Autodesk Fusion 360 part; units mm, degrees
(part 6 of 15)
  spline S4 degree 5 poles (-14.2309, -4.8539) (-14.231, -4.8539) (-14.2312, -4.854) (-14.2315, -4.8541) (-14.232, -4.8543) (-14.2328, -4.8546) (-14.2336, -4.8549) (-14.2346, -4.8552) (-14.2356, -4.8556) (-14.2368, -4.8561) (-14.2381, -4.8566) (-14.2395, -4.8571) (-14.241, -4.8577) (-14.2426, -4.8583) (-14.2443, -4.8589) (-14.2461, -4.8596) (-14.2479, -4.8604) (-14.2499, -4.8612) (-14.252, -4.862) (-14.2542, -4.8629) (-14.2564, -4.8638) (-14.2588, -4.8648) (-14.2612, -4.8658) (-14.2637, -4.8669) (-14.2663, -4.868) (-14.269, -4.8691) (-14.2718, -4.8703) (-14.2747, -4.8715) (-14.2776, -4.8728) (-14.2807, -4.8741) (-14.2838, -4.8755) (-14.2869, -4.8769) (-14.2902, -4.8784) (-14.2935, -4.8799) (-14.2969, -4.8814) (-14.3004, -4.883) (-14.304, -4.8846) (-14.3076, -4.8863) (-14.3113, -4.888) (-14.3151, -4.8898) (-14.319, -4.8916) (-14.3229, -4.8935) (-14.3269, -4.8954) (-14.3309, -4.8973) (-14.335, -4.8993) (-14.3392, -4.9014) (-14.3435, -4.9035) (-14.3478, -4.9056) (-14.3521, -4.9078) (-14.3566, -4.91) (-14.3611, -4.9122) (-14.3656, -4.9145) (-14.3703, -4.9169) (-14.375, -4.9193) (-14.3797, -4.9217) (-14.3845, -4.9242) (-14.3894, -4.9268) (-14.3943, -4.9293) (-14.3992, -4.932) (-14.4043, -4.9346) (-14.4094, -4.9373) (-14.4145, -4.9401) (-14.4197, -4.9429) (-14.4249, -4.9457) (-14.4302, -4.9486) (-14.4356, -4.9516) (-14.441, -4.9545) (-14.4465, -4.9576) (-14.452, -4.9606) (-14.4575, -4.9637) (-14.4631, -4.9669) (-14.4688, -4.9701) (-14.4745, -4.9734) (-14.4802, -4.9766) (-14.486, -4.98) (-14.4919, -4.9834) (-14.4978, -4.9868) (-14.5037, -4.9903) (-14.5097, -4.9938) (-14.5157, -4.9974) (-14.5218, -5.001) (-14.5279, -5.0046) (-14.534, -5.0083) (-14.5402, -5.0121) (-14.5465, -5.0158) (-14.5528, -5.0197) (-14.5591, -5.0235) (-14.5655, -5.0275) (-14.5719, -5.0314) (-14.5783, -5.0354) (-14.5848, -5.0395) (-14.5913, -5.0436) (-14.5979, -5.0477) (-14.6045, -5.0519) (-14.6111, -5.0562) (-14.6178, -5.0604) (-14.6245, -5.0648) (-14.6313, -5.0691) (-14.6381, -5.0735) (-14.6449, -5.078) (-14.6518, -5.0825) (-14.6587, -5.087) (-14.6656, -5.0916) (-14.6726, -5.0963) (-14.6796, -5.1009) (-14.6866, -5.1057) (-14.6937, -5.1104) (-14.7008, -5.1152) (-14.7079, -5.1201) (-14.7151, -5.125) (-14.7223, -5.1299) (-14.7295, -5.1349) (-14.7368, -5.14) (-14.7441, -5.145) (-14.7514, -5.1502) (-14.7587, -5.1553) (-14.7661, -5.1605) (-14.7735, -5.1658) (-14.781, -5.1711) (-14.7884, -5.1764) (-14.7959, -5.1818) (-14.8035, -5.1873) (-14.811, -5.1927) (-14.8186, -5.1982) (-14.8262, -5.2038) (-14.8338, -5.2094) (-14.8415, -5.2151) (-14.8492, -5.2208) (-14.8569, -5.2265) (-14.8646, -5.2323) (-14.8724, -5.2381) (-14.8802, -5.244) (-14.888, -5.2499) (-14.8959, -5.2559) (-14.9037, -5.2619) (-14.9116, -5.2679) (-14.9195, -5.274) (-14.9275, -5.2801) (-14.9354, -5.2863) (-14.9434, -5.2925) (-14.9514, -5.2988) (-14.9594, -5.3051) (-14.9675, -5.3114) (-14.9755, -5.3178) (-14.9836, -5.3243) (-14.9918, -5.3308) (-14.9999, -5.3373) (-15.008, -5.3439) (-15.0162, -5.3505) (-15.0244, -5.3571) (-15.0326, -5.3638) (-15.0409, -5.3706) (-15.0491, -5.3773) (-15.0574, -5.3842) (-15.0657, -5.391) (-15.074, -5.398) (-15.0823, -5.4049) (-15.0907, -5.4119) (-15.099, -5.419) (-15.1074, -5.426) (-15.1158, -5.4332) (-15.1242, -5.4403) (-15.1327, -5.4476) (-15.1411, -5.4548) (-15.1496, -5.4621) (-15.1581, -5.4695) (-15.1666, -5.4769) (-15.1751, -5.4843) (-15.1836, -5.4918) (-15.1922, -5.4993) (-15.2008, -5.5068) (-15.2093, -5.5144) (-15.2179, -5.5221) (-15.2265, -5.5298) (-15.2352, -5.5375) (-15.2438, -5.5453) (-15.2524, -5.5531) (-15.2611, -5.5609) (-15.2698, -5.5688) (-15.2785, -5.5768) (-15.2872, -5.5848) (-15.2959, -5.5928) (-15.3046, -5.6008) (-15.3134, -5.609) (-15.3221, -5.6171) (-15.3309, -5.6253) (-15.3397, -5.6335) (-15.3484, -5.6418) (-15.3572, -5.6501) (-15.3661, -5.6585) (-15.3749, -5.6669) (-15.3837, -5.6753) (-15.3926, -5.6838) (-15.4014, -5.6924) (-15.4103, -5.7009) (-15.4192, -5.7096) (-15.428, -5.7182) (-15.4369, -5.7269) (-15.4458, -5.7356) (-15.4548, -5.7444) (-15.4637, -5.7532) (-15.4726, -5.7621) (-15.4816, -5.771) (-15.4905, -5.78) (-15.4995, -5.789) (-15.5084, -5.798) (-15.5174, -5.8071) (-15.5264, -5.8162) (-15.5354, -5.8253) (-15.5444, -5.8345) (-15.5534, -5.8437) (-15.5624, -5.853) (-15.5714, -5.8623) (-15.5804, -5.8717) (-15.5895, -5.8811) (-15.5985, -5.8905) (-15.6075, -5.9) (-15.6166, -5.9096) (-15.6256, -5.9191) (-15.6347, -5.9287) (-15.6438, -5.9384) (-15.6529, -5.9481) (-15.6619, -5.9578) (-15.671, -5.9676) (-15.6801, -5.9774) (-15.6892, -5.9872) (-15.6983, -5.9971) (-15.7074, -6.007) (-15.7165, -6.017) (-15.7256, -6.027) (-15.7347, -6.0371) (-15.7439, -6.0472) (-15.753, -6.0573) (-15.7621, -6.0675) (-15.7712, -6.0777) (-15.7804, -6.0879) (-15.7895, -6.0982) (-15.7986, -6.1086) (-15.8078, -6.1189) (-15.8169, -6.1293) (-15.8261, -6.1398) (-15.8334, -6.1482) (-15.8389, -6.1545) (-15.8425, -6.1587) (-15.8444, -6.1608) knots 0 0 0 0 0 0 0.00416667 0.00833333 0.0125 0.01666667 0.02083333 0.025 0.02916667 0.03333333 0.0375 0.04166667 0.04583333 0.05 0.05416667 0.05833333 0.0625 0.06666667 0.07083333 0.075 0.07916667 0.08333333 0.0875 0.09166667 0.09583333 0.1 0.10416667 0.10833333 0.1125 0.11666667 0.12083333 0.125 0.12916667 0.13333333 0.1375 0.14166667 0.14583333 0.15 0.15416667 0.15833333 0.1625 0.16666667 0.17083333 0.175 0.17916667 0.18333333 0.1875 0.19166667 0.19583333 0.2 0.20416667 0.20833333 0.2125 0.21666667 0.22083333 0.225 0.22916667 0.23333333 0.2375 0.24166667 0.24583333 0.25 0.25416667 0.25833333 0.2625 0.26666667 0.27083333 0.275 0.27916667 0.28333333 0.2875 0.29166667 0.29583333 0.3 0.30416667 0.30833333 0.3125 0.31666667 0.32083333 0.325 0.32916667 0.33333333 0.3375 0.34166667 0.34583333 0.35 0.35416667 0.35833333 0.3625 0.36666667 0.37083333 0.375 0.37916667 0.38333333 0.3875 0.39166667 0.39583333 0.4 0.40416667 0.40833333 0.4125 0.41666667 0.42083333 0.425 0.42916667 0.43333333 0.4375 0.44166667 0.44583333 0.45 0.45416667 0.45833333 0.4625 0.46666667 0.47083333 0.475 0.47916667 0.48333333 0.4875 0.49166667 0.49583333 0.5 0.50416667 0.50833333 0.5125 0.51666667 0.52083333 0.525 0.52916667 0.53333333 0.5375 0.54166667 0.54583333 0.55 0.55416667 0.55833333 0.5625 0.56666667 0.57083333 0.575 0.57916667 0.58333333 0.5875 0.59166667 0.59583333 0.6 0.60416667 0.60833333 0.6125 0.61666667 0.62083333 0.625 0.62916667 0.63333333 0.6375 0.64166667 0.64583333 0.65 0.65416667 0.65833333 0.6625 0.66666667 0.67083333 0.675 0.67916667 0.68333333 0.6875 0.69166667 0.69583333 0.7 0.70416667 0.70833333 0.7125 0.71666667 0.72083333 0.725 0.72916667 0.73333333 0.7375 0.74166667 0.74583333 0.75 0.75416667 0.75833333 0.7625 0.76666667 0.77083333 0.775 0.77916667 0.78333333 0.7875 0.79166667 0.79583333 0.8 0.80416667 0.80833333 0.8125 0.81666667 0.82083333 0.825 0.82916667 0.83333333 0.8375 0.84166667 0.84583333 0.85 0.85416667 0.85833333 0.8625 0.86666667 0.87083333 0.875 0.87916667 0.88333333 0.8875 0.89166667 0.89583333 0.9 0.90416667 0.90833333 0.9125 0.91666667 0.92083333 0.925 0.92916667 0.93333333 0.9375 0.94166667 0.94583333 0.95 0.95416667 0.95833333 0.9625 0.96666667 0.97083333 0.975 0.97916667 0.98333333 0.9875 0.99166667 0.99583333 1 1 1 1 1 1
  arc A5 (-15.8444, -6.1608) -> (-15.56, -6.8473) centre (0, 0) ccw
  spline S5 degree 5 poles (-15.56, -6.8473) (-15.5572, -6.8475) (-15.5517, -6.8479) (-15.5433, -6.8485) (-15.5322, -6.8492) (-15.5184, -6.8502) (-15.5045, -6.851) (-15.4907, -6.8519) (-15.477, -6.8528) (-15.4632, -6.8536) (-15.4495, -6.8544) (-15.4358, -6.8551) (-15.4222, -6.8559) (-15.4086, -6.8566) (-15.395, -6.8573) (-15.3814, -6.8579) (-15.3679, -6.8586) (-15.3544, -6.8592) (-15.341, -6.8598) (-15.3275, -6.8603) (-15.3141, -6.8609) (-15.3008, -6.8614) (-15.2874, -6.8619) (-15.2741, -6.8623) (-15.2609, -6.8628) (-15.2476, -6.8632) (-15.2344, -6.8636) (-15.2213, -6.8639) (-15.2081, -6.8642) (-15.195, -6.8646) (-15.182, -6.8648) (-15.1689, -6.8651) (-15.1559, -6.8653) (-15.143, -6.8656) (-15.13, -6.8657) (-15.1171, -6.8659) (-15.1043, -6.866) (-15.0915, -6.8662) (-15.0787, -6.8663) (-15.0659, -6.8663) (-15.0532, -6.8664) (-15.0405, -6.8664) (-15.0278, -6.8664) (-15.0152, -6.8664) (-15.0026, -6.8663) (-14.9901, -6.8662) (-14.9776, -6.8661) (-14.9651, -6.866) (-14.9527, -6.8659) (-14.9403, -6.8657) (-14.9279, -6.8655) (-14.9156, -6.8653) (-14.9033, -6.8651) (-14.891, -6.8649) (-14.8788, -6.8646) (-14.8666, -6.8643) (-14.8545, -6.864) (-14.8424, -6.8636) (-14.8303, -6.8633) (-14.8183, -6.8629) (-14.8063, -6.8625) (-14.7943, -6.8621) (-14.7824, -6.8616) (-14.7705, -6.8611) (-14.7587, -6.8606) (-14.7469, -6.8601) (-14.7351, -6.8596) (-14.7234, -6.8591) (-14.7117, -6.8585) (-14.7001, -6.8579) (-14.6885, -6.8573) (-14.6769, -6.8567) (-14.6654, -6.856) (-14.6539, -6.8553) (-14.6425, -6.8546) (-14.6311, -6.8539) (-14.6197, -6.8532) (-14.6084, -6.8524) (-14.5971, -6.8517) (-14.5859, -6.8509) (-14.5747, -6.8501) (-14.5635, -6.8493) (-14.5524, -6.8484) (-14.5414, -6.8475) (-14.5303, -6.8467) (-14.5194, -6.8458) (-14.5084, -6.8449) (-14.4975, -6.8439) (-14.4867, -6.843) (-14.4759, -6.842) (-14.4651, -6.841) (-14.4544, -6.84) (-14.4437, -6.839) (-14.4331, -6.8379) (-14.4225, -6.8369) (-14.4119, -6.8358) (-14.4014, -6.8347) (-14.391, -6.8336) (-14.3805, -6.8325) (-14.3702, -6.8314) (-14.3599, -6.8302) (-14.3496, -6.829) (-14.3394, -6.8278) (-14.3292, -6.8266) (-14.319, -6.8254) (-14.309, -6.8242) (-14.2989, -6.823) (-14.2889, -6.8217) (-14.279, -6.8204) (-14.2691, -6.8191) (-14.2592, -6.8178) (-14.2494, -6.8165) (-14.2397, -6.8152) (-14.2299, -6.8138) (-14.2203, -6.8125) (-14.2107, -6.8111) (-14.2011, -6.8097) (-14.1916, -6.8083) (-14.1821, -6.8069) (-14.1727, -6.8055) (-14.1634, -6.8041) (-14.154, -6.8026) (-14.1448, -6.8011) (-14.1356, -6.7997) (-14.1264, -6.7982) (-14.1173, -6.7967) (-14.1082, -6.7952) (-14.0992, -6.7937) (-14.0903, -6.7922) (-14.0814, -6.7906) (-14.0725, -6.7891) (-14.0637, -6.7875) (-14.055, -6.786) (-14.0463, -6.7844) (-14.0376, -6.7828) (-14.0291, -6.7812) (-14.0205, -6.7796) (-14.012, -6.778) (-14.0036, -6.7764) (-13.9953, -6.7747) (-13.9869, -6.7731) (-13.9787, -6.7715) (-13.9705, -6.7698) (-13.9623, -6.7682) (-13.9542, -6.7665) (-13.9462, -6.7648) (-13.9382, -6.7632) (-13.9303, -6.7615) (-13.9224, -6.7598) (-13.9146, -6.7581) (-13.9069, -6.7564) (-13.8992, -6.7547) (-13.8916, -6.753) (-13.884, -6.7513) (-13.8765, -6.7496) (-13.869, -6.7478) (-13.8616, -6.7461) (-13.8543, -6.7444) (-13.847, -6.7427) (-13.8398, -6.7409) (-13.8327, -6.7392) (-13.8256, -6.7374) (-13.8185, -6.7357) (-13.8116, -6.734) (-13.8047, -6.7322) (-13.7978, -6.7305) (-13.791, -6.7287) (-13.7843, -6.727) (-13.7777, -6.7253) (-13.7711, -6.7235) (-13.7645, -6.7218) (-13.7581, -6.72) (-13.7517, -6.7183) (-13.7454, -6.7166) (-13.7391, -6.7148) (-13.7329, -6.7131) (-13.7268, -6.7114) (-13.7207, -6.7097) (-13.7147, -6.7079) (-13.7088, -6.7062) (-13.7029, -6.7045) (-13.6971, -6.7028) (-13.6914, -6.7011) (-13.6858, -6.6994) (-13.6802, -6.6977) (-13.6747, -6.6961) (-13.6692, -6.6944) (-13.6639, -6.6927) (-13.6586, -6.6911) (-13.6533, -6.6894) (-13.6482, -6.6878) (-13.6431, -6.6862) (-13.6381, -6.6845) (-13.6332, -6.6829) (-13.6283, -6.6813) (-13.6235, -6.6798) (-13.6188, -6.6782) (-13.6142, -6.6766) (-13.6096, -6.6751) (-13.6051, -6.6736) (-13.6007, -6.672) (-13.5964, -6.6705) (-13.5922, -6.669) (-13.588, -6.6676) (-13.5839, -6.6661) (-13.5799, -6.6647) (-13.576, -6.6633) (-13.5722, -6.6619) (-13.5684, -6.6605) (-13.5647, -6.6591) (-13.5611, -6.6578) (-13.5576, -6.6565) (-13.5542, -6.6552) (-13.5509, -6.6539) (-13.5476, -6.6526) (-13.5445, -6.6514) (-13.5414, -6.6502) (-13.5384, -6.649) (-13.5355, -6.6479) (-13.5327, -6.6468) (-13.53, -6.6457) (-13.5274, -6.6446) (-13.5248, -6.6436) (-13.5224, -6.6426) (-13.5201, -6.6416) (-13.5178, -6.6406) (-13.5156, -6.6397) (-13.5136, -6.6389) (-13.5116, -6.638) (-13.5098, -6.6372) (-13.508, -6.6364) (-13.5063, -6.6357) (-13.5048, -6.635) (-13.5033, -6.6344) (-13.502, -6.6338) (-13.5007, -6.6332) (-13.4996, -6.6327) (-13.4985, -6.6322) (-13.4976, -6.6318) (-13.4968, -6.6314) (-13.4961, -6.6311) (-13.4956, -6.6308) (-13.4953, -6.6307) (-13.4951, -6.6306) (-13.495, -6.6306) knots -1 -1 -1 -1 -1 -1 -0.99583333 -0.99166667 -0.9875 -0.98333333 -0.97916667 -0.975 -0.97083333 -0.96666667 -0.9625 -0.95833333 -0.95416667 -0.95 -0.94583333 -0.94166667 -0.9375 -0.93333333 -0.92916667 -0.925 -0.92083333 -0.91666667 -0.9125 -0.90833333 -0.90416667 -0.9 -0.89583333 -0.89166667 -0.8875 -0.88333333 -0.87916667 -0.875 -0.87083333 -0.86666667 -0.8625 -0.85833333 -0.85416667 -0.85 -0.84583333 -0.84166667 -0.8375 -0.83333333 -0.82916667 -0.825 -0.82083333 -0.81666667 -0.8125 -0.80833333 -0.80416667 -0.8 -0.79583333 -0.79166667 -0.7875 -0.78333333 -0.77916667 -0.775 -0.77083333 -0.76666667 -0.7625 -0.75833333 -0.75416667 -0.75 -0.74583333 -0.74166667 -0.7375 -0.73333333 -0.72916667 -0.725 -0.72083333 -0.71666667 -0.7125 -0.70833333 -0.70416667 -0.7 -0.69583333 -0.69166667 -0.6875 -0.68333333 -0.67916667 -0.675 -0.67083333 -0.66666667 -0.6625 -0.65833333 -0.65416667 -0.65 -0.64583333 -0.64166667 -0.6375 -0.63333333 -0.62916667 -0.625 -0.62083333 -0.61666667 -0.6125 -0.60833333 -0.60416667 -0.6 -0.59583333 -0.59166667 -0.5875 -0.58333333 -0.57916667 -0.575 -0.57083333 -0.56666667 -0.5625 -0.55833333 -0.55416667 -0.55 -0.54583333 -0.54166667 -0.5375 -0.53333333 -0.52916667 -0.525 -0.52083333 -0.51666667 -0.5125 -0.50833333 -0.50416667 -0.5 -0.49583333 -0.49166667 -0.4875 -0.48333333 -0.47916667 -0.475 -0.47083333 -0.46666667 -0.4625 -0.45833333 -0.45416667 -0.45 -0.44583333 -0.44166667 -0.4375 -0.43333333 -0.42916667 -0.425 -0.42083333 -0.41666667 -0.4125 -0.40833333 -0.40416667 -0.4 -0.39583333 -0.39166667 -0.3875 -0.38333333 -0.37916667 -0.375 -0.37083333 -0.36666667 -0.3625 -0.35833333 -0.35416667 -0.35 -0.34583333 -0.34166667 -0.3375 -0.33333333 -0.32916667 -0.325 -0.32083333 -0.31666667 -0.3125 -0.30833333 -0.30416667 -0.3 -0.29583333 -0.29166667 -0.2875 -0.28333333 -0.27916667 -0.275 -0.27083333 -0.26666667 -0.2625 -0.25833333 -0.25416667 -0.25 -0.24583333 -0.24166667 -0.2375 -0.23333333 -0.22916667 -0.225 -0.22083333 -0.21666667 -0.2125 -0.20833333 -0.20416667 -0.2 -0.19583333 -0.19166667 -0.1875 -0.18333333 -0.17916667 -0.175 -0.17083333 -0.16666667 -0.1625 -0.15833333 -0.15416667 -0.15 -0.14583333 -0.14166667 -0.1375 -0.13333333 -0.12916667 -0.125 -0.12083333 -0.11666667 -0.1125 -0.10833333 -0.10416667 -0.1 -0.09583333 -0.09166667 -0.0875 -0.08333333 -0.07916667 -0.075 -0.07083333 -0.06666667 -0.0625 -0.05833333 -0.05416667 -0.05 -0.04583333 -0.04166667 -0.0375 -0.03333333 -0.02916667 -0.025 -0.02083333 -0.01666667 -0.0125 -0.00833333 -0.00416667 0 0 0 0 0 0
  line L10 (-13.495, -6.6306) -> (-13.4942, -6.6302)
  line L11 (-13.4942, -6.6302) -> (-13.2384, -6.5045)
  arc A6 (-13.2384, -6.5045) -> (-12.7631, -7.3936) centre (0, 0) ccw
  line L12 (-12.7631, -7.3936) -> (-13.0098, -7.5365)
  line L13 (-13.0098, -7.5365) -> (-13.0105, -7.537)
  spline S6 degree 5 poles (-13.0105, -7.537) (-13.0106, -7.537) (-13.0108, -7.5371) (-13.0111, -7.5373) (-13.0115, -7.5376) (-13.0122, -7.538) (-13.013, -7.5384) (-13.0139, -7.539) (-13.0148, -7.5396) (-13.0159, -7.5402) (-13.0171, -7.541) (-13.0183, -7.5417) (-13.0197, -7.5426) (-13.0211, -7.5435) (-13.0226, -7.5445) (-13.0243, -7.5455) (-13.026, -7.5466) (-13.0278, -7.5478) (-13.0296, -7.549) (-13.0316, -7.5503) (-13.0336, -7.5516) (-13.0357, -7.5531) (-13.0379, -7.5545) (-13.0402, -7.5561) (-13.0425, -7.5576) (-13.045, -7.5593) (-13.0474, -7.561) (-13.05, -7.5628) (-13.0526, -7.5646) (-13.0554, -7.5665) (-13.0581, -7.5684) (-13.061, -7.5704) (-13.0639, -7.5725) (-13.0669, -7.5746) (-13.0699, -7.5768) (-13.073, -7.5791) (-13.0762, -7.5814) (-13.0794, -7.5837) (-13.0827, -7.5861) (-13.0861, -7.5886) (-13.0895, -7.5911) (-13.093, -7.5937) (-13.0965, -7.5964) (-13.1001, -7.5991) (-13.1038, -7.6018) (-13.1075, -7.6046) (-13.1112, -7.6075) (-13.115, -7.6104) (-13.1189, -7.6134) (-13.1228, -7.6165) (-13.1268, -7.6196) (-13.1308, -7.6227) (-13.1349, -7.6259) (-13.139, -7.6292) (-13.1432, -7.6325) (-13.1474, -7.6359) (-13.1517, -7.6393) (-13.156, -7.6428) (-13.1604, -7.6463) (-13.1648, -7.6499) (-13.1693, -7.6536) (-13.1738, -7.6573) (-13.1783, -7.6611) (-13.1829, -7.6649) (-13.1875, -7.6687) (-13.1922, -7.6727) (-13.1969, -7.6766) (-13.2017, -7.6807) (-13.2065, -7.6847) (-13.2113, -7.6889) (-13.2162, -7.6931) (-13.2211, -7.6973) (-13.2261, -7.7016) (-13.2311, -7.706) (-13.2361, -7.7104) (-13.2412, -7.7148) (-13.2463, -7.7194) (-13.2515, -7.7239) (-13.2566, -7.7285) (-13.2618, -7.7332) (-13.2671, -7.7379) (-13.2724, -7.7427) (-13.2777, -7.7475) (-13.2831, -7.7524) (-13.2884, -7.7573) (-13.2939, -7.7623) (-13.2993, -7.7674) (-13.3048, -7.7724) (-13.3103, -7.7776) (-13.3158, -7.7828) (-13.3214, -7.788) (-13.327, -7.7933) (-13.3326, -7.7987) (-13.3383, -7.8041) (-13.344, -7.8095) (-13.3497, -7.815) (-13.3555, -7.8206) (-13.3612, -7.8262) (-13.367, -7.8318) (-13.3728, -7.8375) (-13.3787, -7.8433) (-13.3846, -7.8491) (-13.3905, -7.8549) (-13.3964, -7.8608) (-13.4024, -7.8668) (-13.4083, -7.8728) (-13.4143, -7.8788) (-13.4204, -7.8849) (-13.4264, -7.8911) (-13.4325, -7.8973) (-13.4386, -7.9035) (-13.4447, -7.9099) (-13.4508, -7.9162) (-13.457, -7.9226) (-13.4632, -7.9291) (-13.4694, -7.9356) (-13.4756, -7.9421) (-13.4819, -7.9487) (-13.4881, -7.9554) (-13.4944, -7.9621) (-13.5007, -7.9688) (-13.507, -7.9756) (-13.5134, -7.9824) (-13.5197, -7.9893) (-13.5261, -7.9963) (-13.5325, -8.0033) (-13.5389, -8.0103) (-13.5453, -8.0174) (-13.5518, -8.0245) (-13.5583, -8.0317) (-13.5647, -8.0389) (-13.5712, -8.0462) (-13.5777, -8.0535) (-13.5843, -8.0609) (-13.5908, -8.0683) (-13.5974, -8.0758) (-13.6039, -8.0833) (-13.6105, -8.0909) (-13.6171, -8.0985) (-13.6237, -8.1061) (-13.6304, -8.1138) (-13.637, -8.1216) (-13.6437, -8.1294) (-13.6503, -8.1372) (-13.657, -8.1451) (-13.6637, -8.1531) (-13.6704, -8.1611) (-13.6771, -8.1691) (-13.6839, -8.1772) (-13.6906, -8.1853) (-13.6973, -8.1935) (-13.7041, -8.2017) (-13.7109, -8.21) (-13.7177, -8.2183) (-13.7245, -8.2266) (-13.7313, -8.235) (-13.7381, -8.2435) (-13.7449, -8.252) (-13.7517, -8.2605) (-13.7586, -8.2691) (-13.7654, -8.2777) (-13.7723, -8.2864) (-13.7791, -8.2951) (-13.786, -8.3039) (-13.7929, -8.3127) (-13.7998, -8.3216) (-13.8067, -8.3305) (-13.8136, -8.3394) (-13.8205, -8.3484) (-13.8274, -8.3575) (-13.8343, -8.3665) (-13.8413, -8.3757) (-13.8482, -8.3848) (-13.8552, -8.3941) (-13.8621, -8.4033) (-13.8691, -8.4126) (-13.876, -8.422) (-13.883, -8.4314) (-13.89, -8.4408) (-13.8969, -8.4503) (-13.9039, -8.4598) (-13.9109, -8.4694) (-13.9179, -8.479) (-13.9249, -8.4887) (-13.9319, -8.4984) (-13.9389, -8.5081) (-13.9459, -8.5179) (-13.9529, -8.5277) (-13.9599, -8.5376) (-13.9669, -8.5475) (-13.9739, -8.5575) (-13.9809, -8.5675) (-13.9879, -8.5776) (-13.995, -8.5877) (-14.002, -8.5978) (-14.009, -8.608) (-14.016, -8.6182) (-14.0231, -8.6285) (-14.0301, -8.6388) (-14.0371, -8.6491) (-14.0441, -8.6595) (-14.0512, -8.67) (-14.0582, -8.6804) (-14.0652, -8.6909) (-14.0723, -8.7015) (-14.0793, -8.7121) (-14.0863, -8.7228) (-14.0934, -8.7335) (-14.1004, -8.7442) (-14.1074, -8.755) (-14.1145, -8.7658) (-14.1215, -8.7766) (-14.1285, -8.7875) (-14.1355, -8.7985) (-14.1426, -8.8095) (-14.1496, -8.8205) (-14.1566, -8.8315) (-14.1636, -8.8426) (-14.1706, -8.8538) (-14.1777, -8.865) (-14.1847, -8.8762) (-14.1917, -8.8875) (-14.1987, -8.8988) (-14.2057, -8.9101) (-14.2127, -8.9215) (-14.2197, -8.933) (-14.2267, -8.9445) (-14.2337, -8.956) (-14.2407, -8.9675) (-14.2476, -8.9791) (-14.2546, -8.9908) (-14.2616, -9.0024) (-14.2686, -9.0142) (-14.2755, -9.0259) (-14.2825, -9.0377) (-14.2895, -9.0495) (-14.2964, -9.0614) (-14.3033, -9.0733) (-14.3103, -9.0853) (-14.3172, -9.0973) (-14.3242, -9.1093) (-14.3297, -9.119) (-14.3339, -9.1263) (-14.3366, -9.1311) (-14.338, -9.1335) knots 0 0 0 0 0 0 0.00416667 0.00833333 0.0125 0.01666667 0.02083333 0.025 0.02916667 0.03333333 0.0375 0.04166667 0.04583333 0.05 0.05416667 0.05833333 0.0625 0.06666667 0.07083333 0.075 0.07916667 0.08333333 0.0875 0.09166667 0.09583333 0.1 0.10416667 0.10833333 0.1125 0.11666667 0.12083333 0.125 0.12916667 0.13333333 0.1375 0.14166667 0.14583333 0.15 0.15416667 0.15833333 0.1625 0.16666667 0.17083333 0.175 0.17916667 0.18333333 0.1875 0.19166667 0.19583333 0.2 0.20416667 0.20833333 0.2125 0.21666667 0.22083333 0.225 0.22916667 0.23333333 0.2375 0.24166667 0.24583333 0.25 0.25416667 0.25833333 0.2625 0.26666667 0.27083333 0.275 0.27916667 0.28333333 0.2875 0.29166667 0.29583333 0.3 0.30416667 0.30833333 0.3125 0.31666667 0.32083333 0.325 0.32916667 0.33333333 0.3375 0.34166667 0.34583333 0.35 0.35416667 0.35833333 0.3625 0.36666667 0.37083333 0.375 0.37916667 0.38333333 0.3875 0.39166667 0.39583333 0.4 0.40416667 0.40833333 0.4125 0.41666667 0.42083333 0.425 0.42916667 0.43333333 0.4375 0.44166667 0.44583333 0.45 0.45416667 0.45833333 0.4625 0.46666667 0.47083333 0.475 0.47916667 0.48333333 0.4875 0.49166667 0.49583333 0.5 0.50416667 0.50833333 0.5125 0.51666667 0.52083333 0.525 0.52916667 0.53333333 0.5375 0.54166667 0.54583333 0.55 0.55416667 0.55833333 0.5625 0.56666667 0.57083333 0.575 0.57916667 0.58333333 0.5875 0.59166667 0.59583333 0.6 0.60416667 0.60833333 0.6125 0.61666667 0.62083333 0.625 0.62916667 0.63333333 0.6375 0.64166667 0.64583333 0.65 0.65416667 0.65833333 0.6625 0.66666667 0.67083333 0.675 0.67916667 0.68333333 0.6875 0.69166667 0.69583333 0.7 0.70416667 0.70833333 0.7125 0.71666667 0.72083333 0.725 0.72916667 0.73333333 0.7375 0.74166667 0.74583333 0.75 0.75416667 0.75833333 0.7625 0.76666667 0.77083333 0.775 0.77916667 0.78333333 0.7875 0.79166667 0.79583333 0.8 0.80416667 0.80833333 0.8125 0.81666667 0.82083333 0.825 0.82916667 0.83333333 0.8375 0.84166667 0.84583333 0.85 0.85416667 0.85833333 0.8625 0.86666667 0.87083333 0.875 0.87916667 0.88333333 0.8875 0.89166667 0.89583333 0.9 0.90416667 0.90833333 0.9125 0.91666667 0.92083333 0.925 0.92916667 0.93333333 0.9375 0.94166667 0.94583333 0.95 0.95416667 0.95833333 0.9625 0.96666667 0.97083333 0.975 0.97916667 0.98333333 0.9875 0.99166667 0.99583333 1 1 1 1 1 1
  arc A7 (-14.338, -9.1335) -> (-13.9252, -9.7513) centre (0, 0) ccw
  spline S7 degree 5 poles (-13.9252, -9.7513) (-13.9224, -9.751) (-13.9169, -9.7503) (-13.9086, -9.7492) (-13.8975, -9.7478) (-13.8838, -9.746) (-13.87, -9.7442) (-13.8563, -9.7424) (-13.8427, -9.7405) (-13.829, -9.7386) (-13.8154, -9.7367) (-13.8019, -9.7348) (-13.7883, -9.7329) (-13.7748, -9.7309) (-13.7614, -9.7289) (-13.748, -9.7269) (-13.7346, -9.7249) (-13.7212, -9.7229) (-13.7079, -9.7208) (-13.6946, -9.7188) (-13.6814, -9.7167) (-13.6682, -9.7146) (-13.655, -9.7125) (-13.6419, -9.7103) (-13.6288, -9.7081) (-13.6157, -9.706) (-13.6027, -9.7038) (-13.5897, -9.7015) (-13.5768, -9.6993) (-13.5639, -9.6971) (-13.551, -9.6948) (-13.5382, -9.6925) (-13.5254, -9.6902) (-13.5126, -9.6879) (-13.4999, -9.6855) (-13.4872, -9.6832) (-13.4746, -9.6808) (-13.462, -9.6784) (-13.4494, -9.676) (-13.4369, -9.6736) (-13.4244, -9.6712) (-13.4119, -9.6687) (-13.3995, -9.6662) (-13.3871, -9.6637) (-13.3748, -9.6612) (-13.3625, -9.6587) (-13.3503, -9.6562) (-13.3381, -9.6536) (-13.3259, -9.6511) (-13.3137, -9.6485) (-13.3017, -9.6459) (-13.2896, -9.6433) (-13.2776, -9.6407) (-13.2656, -9.638) (-13.2537, -9.6354) (-13.2418, -9.6327) (-13.2299, -9.63) (-13.2181, -9.6273) (-13.2064, -9.6246) (-13.1946, -9.6219) (-13.183, -9.6192) (-13.1713, -9.6164) (-13.1597, -9.6137) (-13.1482, -9.6109) (-13.1367, -9.6081) (-13.1252, -9.6053) (-13.1137, -9.6025) (-13.1024, -9.5997) (-13.091, -9.5968) (-13.0797, -9.594) (-13.0685, -9.5911) (-13.0572, -9.5882) (-13.0461, -9.5853) (-13.0349, -9.5824) (-13.0238, -9.5795) (-13.0128, -9.5766) (-13.0018, -9.5737) (-12.9909, -9.5707) (-12.9799, -9.5678) (-12.9691, -9.5648) (-12.9583, -9.5618) (-12.9475, -9.5589) (-12.9368, -9.5559) (-12.9261, -9.5529) (-12.9154, -9.5498) (-12.9048, -9.5468) (-12.8943, -9.5438) (-12.8838, -9.5407) (-12.8733, -9.5377) (-12.8629, -9.5346) (-12.8525, -9.5316) (-12.8422, -9.5285) (-12.8319, -9.5254) (-12.8217, -9.5223) (-12.8115, -9.5192) (-12.8014, -9.5161) (-12.7913, -9.513) (-12.7813, -9.5098) (-12.7713, -9.5067) (-12.7613, -9.5036) (-12.7514, -9.5004) (-12.7416, -9.4973) (-12.7318, -9.4941) (-12.722, -9.491) (-12.7123, -9.4878) (-12.7027, -9.4846) (-12.6931, -9.4814) (-12.6835, -9.4782) (-12.674, -9.4751) (-12.6645, -9.4719) (-12.6551, -9.4687) (-12.6458, -9.4655) (-12.6365, -9.4622) (-12.6272, -9.459) (-12.618, -9.4558) (-12.6088, -9.4526) (-12.5997, -9.4494) (-12.5907, -9.4461) (-12.5817, -9.4429) (-12.5727, -9.4397) (-12.5638, -9.4364) (-12.555, -9.4332) (-12.5462, -9.43) (-12.5374, -9.4267) (-12.5287, -9.4235) (-12.5201, -9.4203) (-12.5115, -9.417) (-12.5029, -9.4138) (-12.4944, -9.4105) (-12.486, -9.4073) (-12.4776, -9.404) (-12.4693, -9.4008) (-12.461, -9.3976) (-12.4528, -9.3943) (-12.4447, -9.3911) (-12.4365, -9.3878) (-12.4285, -9.3846) (-12.4205, -9.3814) (-12.4125, -9.3781) (-12.4046, -9.3749) (-12.3968, -9.3717) (-12.389, -9.3685) (-12.3813, -9.3652) (-12.3736, -9.362) (-12.366, -9.3588) (-12.3585, -9.3556) (-12.351, -9.3524) (-12.3435, -9.3492) (-12.3362, -9.346) (-12.3288, -9.3428) (-12.3216, -9.3397) (-12.3144, -9.3365) (-12.3072, -9.3333) (-12.3001, -9.3302) (-12.2931, -9.327) (-12.2861, -9.3239) (-12.2792, -9.3208) (-12.2723, -9.3176) (-12.2655, -9.3145) (-12.2588, -9.3114) (-12.2521, -9.3083) (-12.2455, -9.3052) (-12.2389, -9.3021) (-12.2324, -9.2991) (-12.226, -9.296) (-12.2196, -9.293) (-12.2133, -9.2899) (-12.2071, -9.2869) (-12.2009, -9.2839) (-12.1948, -9.2809) (-12.1887, -9.278) (-12.1827, -9.275) (-12.1768, -9.272) (-12.1709, -9.2691) (-12.1651, -9.2662) (-12.1594, -9.2633) (-12.1537, -9.2604) (-12.1481, -9.2575) (-12.1425, -9.2547) (-12.1371, -9.2518) (-12.1316, -9.249) (-12.1263, -9.2462) (-12.121, -9.2434) (-12.1158, -9.2407) (-12.1107, -9.2379) (-12.1056, -9.2352) (-12.1006, -9.2325) (-12.0956, -9.2298) (-12.0907, -9.2272) (-12.0859, -9.2245) (-12.0812, -9.2219) (-12.0765, -9.2193) (-12.0719, -9.2168) (-12.0674, -9.2142) (-12.063, -9.2117) (-12.0586, -9.2092) (-12.0543, -9.2068) (-12.05, -9.2043) (-12.0459, -9.2019) (-12.0418, -9.1996) (-12.0378, -9.1972) (-12.0338, -9.1949) (-12.0299, -9.1926) (-12.0261, -9.1904) (-12.0224, -9.1881) (-12.0188, -9.1859) (-12.0152, -9.1838) (-12.0117, -9.1817) (-12.0083, -9.1796) (-12.005, -9.1775) (-12.0017, -9.1755) (-11.9985, -9.1735) (-11.9954, -9.1716) (-11.9924, -9.1697) (-11.9895, -9.1678) (-11.9866, -9.166) (-11.9838, -9.1642) (-11.9811, -9.1625) (-11.9785, -9.1608) (-11.976, -9.1591) (-11.9735, -9.1575) (-11.9711, -9.156) (-11.9689, -9.1545) (-11.9667, -9.153) (-11.9646, -9.1516) (-11.9625, -9.1502) (-11.9606, -9.1489) (-11.9588, -9.1477) (-11.957, -9.1465) (-11.9553, -9.1453) (-11.9537, -9.1442) (-11.9523, -9.1432) (-11.9509, -9.1422) (-11.9496, -9.1413) (-11.9483, -9.1404) (-11.9472, -9.1396) (-11.9462, -9.1389) (-11.9453, -9.1382) (-11.9445, -9.1376) (-11.9437, -9.1371) (-11.9431, -9.1366) (-11.9427, -9.1363) (-11.9424, -9.1361) (-11.9422, -9.136) (-11.9422, -9.1359) knots -1 -1 -1 -1 -1 -1 -0.99583333 -0.99166667 -0.9875 -0.98333333 -0.97916667 -0.975 -0.97083333 -0.96666667 -0.9625 -0.95833333 -0.95416667 -0.95 -0.94583333 -0.94166667 -0.9375 -0.93333333 -0.92916667 -0.925 -0.92083333 -0.91666667 -0.9125 -0.90833333 -0.90416667 -0.9 -0.89583333 -0.89166667 -0.8875 -0.88333333 -0.87916667 -0.875 -0.87083333 -0.86666667 -0.8625 -0.85833333 -0.85416667 -0.85 -0.84583333 -0.84166667 -0.8375 -0.83333333 -0.82916667 -0.825 -0.82083333 -0.81666667 -0.8125 -0.80833333 -0.80416667 -0.8 -0.79583333 -0.79166667 -0.7875 -0.78333333 -0.77916667 -0.775 -0.77083333 -0.76666667 -0.7625 -0.75833333 -0.75416667 -0.75 -0.74583333 -0.74166667 -0.7375 -0.73333333 -0.72916667 -0.725 -0.72083333 -0.71666667 -0.7125 -0.70833333 -0.70416667 -0.7 -0.69583333 -0.69166667 -0.6875 -0.68333333 -0.67916667 -0.675 -0.67083333 -0.66666667 -0.6625 -0.65833333 -0.65416667 -0.65 -0.64583333 -0.64166667 -0.6375 -0.63333333 -0.62916667 -0.625 -0.62083333 -0.61666667 -0.6125 -0.60833333 -0.60416667 -0.6 -0.59583333 -0.59166667 -0.5875 -0.58333333 -0.57916667 -0.575 -0.57083333 -0.56666667 -0.5625 -0.55833333 -0.55416667 -0.55 -0.54583333 -0.54166667 -0.5375 -0.53333333 -0.52916667 -0.525 -0.52083333 -0.51666667 -0.5125 -0.50833333 -0.50416667 -0.5 -0.49583333 -0.49166667 -0.4875 -0.48333333 -0.47916667 -0.475 -0.47083333 -0.46666667 -0.4625 -0.45833333 -0.45416667 -0.45 -0.44583333 -0.44166667 -0.4375 -0.43333333 -0.42916667 -0.425 -0.42083333 -0.41666667 -0.4125 -0.40833333 -0.40416667 -0.4 -0.39583333 -0.39166667 -0.3875 -0.38333333 -0.37916667 -0.375 -0.37083333 -0.36666667 -0.3625 -0.35833333 -0.35416667 -0.35 -0.34583333 -0.34166667 -0.3375 -0.33333333 -0.32916667 -0.325 -0.32083333 -0.31666667 -0.3125 -0.30833333 -0.30416667 -0.3 -0.29583333 -0.29166667 -0.2875 -0.28333333 -0.27916667 -0.275 -0.27083333 -0.26666667 -0.2625 -0.25833333 -0.25416667 -0.25 -0.24583333 -0.24166667 -0.2375 -0.23333333 -0.22916667 -0.225 -0.22083333 -0.21666667 -0.2125 -0.20833333 -0.20416667 -0.2 -0.19583333 -0.19166667 -0.1875 -0.18333333 -0.17916667 -0.175 -0.17083333 -0.16666667 -0.1625 -0.15833333 -0.15416667 -0.15 -0.14583333 -0.14166667 -0.1375 -0.13333333 -0.12916667 -0.125 -0.12083333 -0.11666667 -0.1125 -0.10833333 -0.10416667 -0.1 -0.09583333 -0.09166667 -0.0875 -0.08333333 -0.07916667 -0.075 -0.07083333 -0.06666667 -0.0625 -0.05833333 -0.05416667 -0.05 -0.04583333 -0.04166667 -0.0375 -0.03333333 -0.02916667 -0.025 -0.02083333 -0.01666667 -0.0125 -0.00833333 -0.00416667 0 0 0 0 0 0
  line L14 (-11.9422, -9.1359) -> (-11.9415, -9.1354)
  line L15 (-11.9415, -9.1354) -> (-11.715, -8.9622)
  arc A8 (-11.715, -8.9622) -> (-11.0754, -9.7415) centre (0, 0) ccw
  line L16 (-11.0754, -9.7415) -> (-11.2895, -9.9298)
  line L17 (-11.2895, -9.9298) -> (-11.2902, -9.9304)
  spline S8 degree 5 poles (-11.2902, -9.9304) (-11.2902, -9.9304) (-11.2904, -9.9306) (-11.2906, -9.9308) (-11.291, -9.9312) (-11.2916, -9.9317) (-11.2923, -9.9323) (-11.293, -9.933) (-11.2939, -9.9338) (-11.2948, -9.9346) (-11.2958, -9.9356) (-11.2969, -9.9366) (-11.298, -9.9377) (-11.2993, -9.9389) (-11.3006, -9.9401) (-11.3019, -9.9414) (-11.3034, -9.9429) (-11.3049, -9.9443) (-11.3065, -9.9459) (-11.3082, -9.9476) (-11.3099, -9.9493) (-11.3117, -9.9511) (-11.3136, -9.9529) (-11.3155, -9.9549) (-11.3175, -9.9569) (-11.3196, -9.959) (-11.3217, -9.9612) (-11.3238, -9.9634) (-11.3261, -9.9657) (-11.3284, -9.9681) (-11.3307, -9.9705) (-11.3331, -9.9731) (-11.3355, -9.9756) (-11.3381, -9.9783) (-11.3406, -9.981) (-11.3432, -9.9838) (-11.3459, -9.9867) (-11.3486, -9.9897) (-11.3514, -9.9927) (-11.3542, -9.9958) (-11.357, -9.9989) (-11.3599, -10.0021) (-11.3629, -10.0054) (-11.3659, -10.0088) (-11.3689, -10.0122) (-11.372, -10.0157) (-11.3751, -10.0192) (-11.3783, -10.0228) (-11.3815, -10.0265) (-11.3848, -10.0303) (-11.3881, -10.0341) (-11.3914, -10.0379) (-11.3948, -10.0419) (-11.3982, -10.0459) (-11.4016, -10.05) (-11.4051, -10.0541) (-11.4086, -10.0583) (-11.4122, -10.0626) (-11.4158, -10.0669) (-11.4194, -10.0713) (-11.4231, -10.0757) (-11.4268, -10.0802) (-11.4305, -10.0848) (-11.4343, -10.0894) (-11.438, -10.0941) (-11.4419, -10.0989) (-11.4457, -10.1037) (-11.4496, -10.1086) (-11.4535, -10.1135) (-11.4575, -10.1186) (-11.4614, -10.1236) (-11.4654, -10.1287) (-11.4694, -10.1339) (-11.4735, -10.1392) (-11.4776, -10.1445) (-11.4817, -10.1498) (-11.4858, -10.1553) (-11.49, -10.1607) (-11.4941, -10.1663) (-11.4984, -10.1719) (-11.5026, -10.1775) (-11.5068, -10.1832) (-11.5111, -10.189) (-11.5154, -10.1948) (-11.5197, -10.2007) (-11.5241, -10.2067) (-11.5284, -10.2127) (-11.5328, -10.2187) (-11.5372, -10.2248) (-11.5416, -10.231) (-11.5461, -10.2373) (-11.5505, -10.2435) (-11.555, -10.2499) (-11.5595, -10.2563) (-11.564, -10.2627) (-11.5686, -10.2692) (-11.5731, -10.2758) (-11.5777, -10.2824) (-11.5823, -10.2891) (-11.5869, -10.2958) (-11.5915, -10.3026) (-11.5961, -10.3094) (-11.6008, -10.3163) (-11.6054, -10.3233) (-11.6101, -10.3303) (-11.6148, -10.3373) (-11.6195, -10.3445) (-11.6242, -10.3516) (-11.629, -10.3588) (-11.6337, -10.3661) (-11.6385, -10.3734) (-11.6432, -10.3808) (-11.648, -10.3882) (-11.6528, -10.3957) (-11.6576, -10.4032) (-11.6624, -10.4108) (-11.6673, -10.4185) (-11.6721, -10.4262) (-11.6769, -10.4339) (-11.6818, -10.4417) (-11.6867, -10.4495) (-11.6915, -10.4574) (-11.6964, -10.4654) (-11.7013, -10.4734) (-11.7062, -10.4814) (-11.7111, -10.4895) (-11.716, -10.4977) (-11.721, -10.5059) (-11.7259, -10.5141) (-11.7308, -10.5225) (-11.7358, -10.5308) (-11.7407, -10.5392) (-11.7457, -10.5477) (-11.7506, -10.5562) (-11.7556, -10.5647) (-11.7606, -10.5733) (-11.7656, -10.582) (-11.7706, -10.5907) (-11.7755, -10.5994) (-11.7805, -10.6082) (-11.7855, -10.6171) (-11.7905, -10.626) (-11.7955, -10.6349) (-11.8006, -10.6439) (-11.8056, -10.653) (-11.8106, -10.6621) (-11.8156, -10.6712) (-11.8206, -10.6804) (-11.8256, -10.6896) (-11.8307, -10.6989) (-11.8357, -10.7083) (-11.8407, -10.7176) (-11.8458, -10.7271) (-11.8508, -10.7365) (-11.8558, -10.7461) (-11.8608, -10.7556) (-11.8659, -10.7652) (-11.8709, -10.7749) (-11.8759, -10.7846) (-11.881, -10.7944) (-11.886, -10.8042) (-11.891, -10.814) (-11.8961, -10.8239) (-11.9011, -10.8339) (-11.9061, -10.8438) (-11.9112, -10.8539) (-11.9162, -10.864) (-11.9212, -10.8741) (-11.9262, -10.8842) (-11.9313, -10.8945) (-11.9363, -10.9047) (-11.9413, -10.915) (-11.9463, -10.9254) (-11.9513, -10.9358) (-11.9563, -10.9462) (-11.9613, -10.9567) (-11.9663, -10.9672) (-11.9713, -10.9778) (-11.9763, -10.9884) (-11.9813, -10.9991) (-11.9863, -11.0098) (-11.9913, -11.0205) (-11.9963, -11.0313) (-12.0012, -11.0422) (-12.0062, -11.053) (-12.0112, -11.064) (-12.0161, -11.0749) (-12.0211, -11.086) (-12.026, -11.097) (-12.031, -11.1081) (-12.0359, -11.1192) (-12.0408, -11.1304) (-12.0458, -11.1417) (-12.0507, -11.1529) (-12.0556, -11.1642) (-12.0605, -11.1756) (-12.0654, -11.187) (-12.0703, -11.1984) (-12.0752, -11.2099) (-12.08, -11.2214) (-12.0849, -11.233) (-12.0898, -11.2446) (-12.0946, -11.2563) (-12.0995, -11.2679) (-12.1043, -11.2797) (-12.1091, -11.2915) (-12.1139, -11.3033) (-12.1188, -11.3151) (-12.1236, -11.327) (-12.1284, -11.339) (-12.1331, -11.3509) (-12.1379, -11.363) (-12.1427, -11.375) (-12.1474, -11.3871) (-12.1522, -11.3993) (-12.1569, -11.4114) (-12.1616, -11.4237) (-12.1664, -11.4359) (-12.1711, -11.4482) (-12.1758, -11.4606) (-12.1805, -11.473) (-12.1851, -11.4854) (-12.1898, -11.4978) (-12.1944, -11.5103) (-12.1991, -11.5229) (-12.2037, -11.5355) (-12.2083, -11.5481) (-12.213, -11.5607) (-12.2176, -11.5734) (-12.2221, -11.5862) (-12.2267, -11.5989) (-12.2313, -11.6118) (-12.2358, -11.6246) (-12.2404, -11.6375) (-12.2449, -11.6504) (-12.2494, -11.6634) (-12.2539, -11.6764) (-12.2584, -11.6894) (-12.2629, -11.7025) (-12.2673, -11.7157) (-12.2718, -11.7288) (-12.2753, -11.7394) (-12.278, -11.7473) (-12.2798, -11.7526) (-12.2806, -11.7552) knots 0 0 0 0 0 0 0.00416667 0.00833333 0.0125 0.01666667 0.02083333 0.025 0.02916667 0.03333333 0.0375 0.04166667 0.04583333 0.05 0.05416667 0.05833333 0.0625 0.06666667 0.07083333 0.075 0.07916667 0.08333333 0.0875 0.09166667 0.09583333 0.1 0.10416667 0.10833333 0.1125 0.11666667 0.12083333 0.125 0.12916667 0.13333333 0.1375 0.14166667 0.14583333 0.15 0.15416667 0.15833333 0.1625 0.16666667 0.17083333 0.175 0.17916667 0.18333333 0.1875 0.19166667 0.19583333 0.2 0.20416667 0.20833333 0.2125 0.21666667 0.22083333 0.225 0.22916667 0.23333333 0.2375 0.24166667 0.24583333 0.25 0.25416667 0.25833333 0.2625 0.26666667 0.27083333 0.275 0.27916667 0.28333333 0.2875 0.29166667 0.29583333 0.3 0.30416667 0.30833333 0.3125 0.31666667 0.32083333 0.325 0.32916667 0.33333333 0.3375 0.34166667 0.34583333 0.35 0.35416667 0.35833333 0.3625 0.36666667 0.37083333 0.375 0.37916667 0.38333333 0.3875 0.39166667 0.39583333 0.4 0.40416667 0.40833333 0.4125 0.41666667 0.42083333 0.425 0.42916667 0.43333333 0.4375 0.44166667 0.44583333 0.45 0.45416667 0.45833333 0.4625 0.46666667 0.47083333 0.475 0.47916667 0.48333333 0.4875 0.49166667 0.49583333 0.5 0.50416667 0.50833333 0.5125 0.51666667 0.52083333 0.525 0.52916667 0.53333333 0.5375 0.54166667 0.54583333 0.55 0.55416667 0.55833333 0.5625 0.56666667 0.57083333 0.575 0.57916667 0.58333333 0.5875 0.59166667 0.59583333 0.6 0.60416667 0.60833333 0.6125 0.61666667 0.62083333 0.625 0.62916667 0.63333333 0.6375 0.64166667 0.64583333 0.65 0.65416667 0.65833333 0.6625 0.66666667 0.67083333 0.675 0.67916667 0.68333333 0.6875 0.69166667 0.69583333 0.7 0.70416667 0.70833333 0.7125 0.71666667 0.72083333 0.725 0.72916667 0.73333333 0.7375 0.74166667 0.74583333 0.75 0.75416667 0.75833333 0.7625 0.76666667 0.77083333 0.775 0.77916667 0.78333333 0.7875 0.79166667 0.79583333 0.8 0.80416667 0.80833333 0.8125 0.81666667 0.82083333 0.825 0.82916667 0.83333333 0.8375 0.84166667 0.84583333 0.85 0.85416667 0.85833333 0.8625 0.86666667 0.87083333 0.875 0.87916667 0.88333333 0.8875 0.89166667 0.89583333 0.9 0.90416667 0.90833333 0.9125 0.91666667 0.92083333 0.925 0.92916667 0.93333333 0.9375 0.94166667 0.94583333 0.95 0.95416667 0.95833333 0.9625 0.96666667 0.97083333 0.975 0.97916667 0.98333333 0.9875 0.99166667 0.99583333 1 1 1 1 1 1
  arc A9 (-12.2806, -11.7552) -> (-11.7552, -12.2806) centre (0, 0) ccw
  spline S9 degree 5 poles (-11.7552, -12.2806) (-11.7526, -12.2798) (-11.7473, -12.278) (-11.7394, -12.2753) (-11.7288, -12.2718) (-11.7157, -12.2673) (-11.7025, -12.2629) (-11.6894, -12.2584) (-11.6764, -12.2539) (-11.6634, -12.2494) (-11.6504, -12.2449) (-11.6375, -12.2404) (-11.6246, -12.2358) (-11.6118, -12.2313) (-11.5989, -12.2267) (-11.5862, -12.2221) (-11.5734, -12.2176) (-11.5607, -12.213) (-11.5481, -12.2083) (-11.5355, -12.2037) (-11.5229, -12.1991) (-11.5103, -12.1944) (-11.4978, -12.1898) (-11.4854, -12.1851) (-11.473, -12.1805) (-11.4606, -12.1758) (-11.4482, -12.1711) (-11.4359, -12.1664) (-11.4237, -12.1616) (-11.4114, -12.1569) (-11.3993, -12.1522) (-11.3871, -12.1474) (-11.375, -12.1427) (-11.363, -12.1379) (-11.3509, -12.1331) (-11.339, -12.1284) (-11.327, -12.1236) (-11.3151, -12.1188) (-11.3033, -12.1139) (-11.2915, -12.1091) (-11.2797, -12.1043) (-11.2679, -12.0995) (-11.2563, -12.0946) (-11.2446, -12.0898) (-11.233, -12.0849) (-11.2214, -12.08) (-11.2099, -12.0752) (-11.1984, -12.0703) (-11.187, -12.0654) (-11.1756, -12.0605) (-11.1642, -12.0556) (-11.1529, -12.0507) (-11.1417, -12.0458) (-11.1304, -12.0408) (-11.1192, -12.0359) (-11.1081, -12.031) (-11.097, -12.026) (-11.086, -12.0211) (-11.0749, -12.0161) (-11.064, -12.0112) (-11.053, -12.0062) (-11.0422, -12.0012) (-11.0313, -11.9963) (-11.0205, -11.9913) (-11.0098, -11.9863) (-10.9991, -11.9813) (-10.9884, -11.9763) (-10.9778, -11.9713) (-10.9672, -11.9663) (-10.9567, -11.9613) (-10.9462, -11.9563) (-10.9358, -11.9513) (-10.9254, -11.9463) (-10.915, -11.9413) (-10.9047, -11.9363) (-10.8945, -11.9313) (-10.8842, -11.9262) (-10.8741, -11.9212) (-10.864, -11.9162) (-10.8539, -11.9112) (-10.8438, -11.9061) (-10.8339, -11.9011) (-10.8239, -11.8961) (-10.814, -11.891) (-10.8042, -11.886) (-10.7944, -11.881) (-10.7846, -11.8759) (-10.7749, -11.8709) (-10.7652, -11.8659) (-10.7556, -11.8608) (-10.7461, -11.8558) (-10.7365, -11.8508) (-10.7271, -11.8458) (-10.7176, -11.8407) (-10.7083, -11.8357) (-10.6989, -11.8307) (-10.6896, -11.8256) (-10.6804, -11.8206) (-10.6712, -11.8156) (-10.6621, -11.8106) (-10.653, -11.8056) (-10.6439, -11.8006) (-10.6349, -11.7955) (-10.626, -11.7905) (-10.6171, -11.7855) (-10.6082, -11.7805) (-10.5994, -11.7755) (-10.5907, -11.7706) (-10.582, -11.7656) (-10.5733, -11.7606) (-10.5647, -11.7556) (-10.5562, -11.7506) (-10.5477, -11.7457) (-10.5392, -11.7407) (-10.5308, -11.7358) (-10.5225, -11.7308) (-10.5141, -11.7259) (-10.5059, -11.721) (-10.4977, -11.716) (-10.4895, -11.7111) (-10.4814, -11.7062) (-10.4734, -11.7013) (-10.4654, -11.6964) (-10.4574, -11.6915) (-10.4495, -11.6867) (-10.4417, -11.6818) (-10.4339, -11.6769) (-10.4262, -11.6721) (-10.4185, -11.6673) (-10.4108, -11.6624) (-10.4032, -11.6576) (-10.3957, -11.6528) (-10.3882, -11.648) (-10.3808, -11.6432) (-10.3734, -11.6385) (-10.3661, -11.6337) (-10.3588, -11.629) (-10.3516, -11.6242) (-10.3445, -11.6195) (-10.3373, -11.6148) (-10.3303, -11.6101) (-10.3233, -11.6054) (-10.3163, -11.6008) (-10.3094, -11.5961) (-10.3026, -11.5915) (-10.2958, -11.5869) (-10.2891, -11.5823) (-10.2824, -11.5777) (-10.2758, -11.5731) (-10.2692, -11.5686) (-10.2627, -11.564) (-10.2563, -11.5595) (-10.2499, -11.555) (-10.2435, -11.5505) (-10.2373, -11.5461) (-10.231, -11.5416) (-10.2248, -11.5372) (-10.2187, -11.5328) (-10.2127, -11.5284) (-10.2067, -11.5241) (-10.2007, -11.5197) (-10.1948, -11.5154) (-10.189, -11.5111) (-10.1832, -11.5068) (-10.1775, -11.5026) (-10.1719, -11.4984) (-10.1663, -11.4941) (-10.1607, -11.49) (-10.1553, -11.4858) (-10.1498, -11.4817) (-10.1445, -11.4776) (-10.1392, -11.4735) (-10.1339, -11.4694) (-10.1287, -11.4654) (-10.1236, -11.4614) (-10.1186, -11.4575) (-10.1135, -11.4535) (-10.1086, -11.4496) (-10.1037, -11.4457) (-10.0989, -11.4419) (-10.0941, -11.438) (-10.0894, -11.4343) (-10.0848, -11.4305) (-10.0802, -11.4268) (-10.0757, -11.4231) (-10.0713, -11.4194) (-10.0669, -11.4158) (-10.0626, -11.4122) (-10.0583, -11.4086) (-10.0541, -11.4051) (-10.05, -11.4016) (-10.0459, -11.3982) (-10.0419, -11.3948) (-10.0379, -11.3914) (-10.0341, -11.3881) (-10.0303, -11.3848) (-10.0265, -11.3815) (-10.0228, -11.3783) (-10.0192, -11.3751) (-10.0157, -11.372) (-10.0122, -11.3689) (-10.0088, -11.3659) (-10.0054, -11.3629) (-10.0021, -11.3599) (-9.9989, -11.357) (-9.9958, -11.3542) (-9.9927, -11.3514) (-9.9897, -11.3486) (-9.9867, -11.3459) (-9.9838, -11.3432) (-9.981, -11.3406) (-9.9783, -11.3381) (-9.9756, -11.3355) (-9.9731, -11.3331) (-9.9705, -11.3307) (-9.9681, -11.3284) (-9.9657, -11.3261) (-9.9634, -11.3238) (-9.9612, -11.3217) (-9.959, -11.3196) (-9.9569, -11.3175) (-9.9549, -11.3155) (-9.9529, -11.3136) (-9.9511, -11.3117) (-9.9493, -11.3099) (-9.9476, -11.3082) (-9.9459, -11.3065) (-9.9443, -11.3049) (-9.9429, -11.3034) (-9.9414, -11.3019) (-9.9401, -11.3006) (-9.9389, -11.2993) (-9.9377, -11.298) (-9.9366, -11.2969) (-9.9356, -11.2958) (-9.9346, -11.2948) (-9.9338, -11.2939) (-9.933, -11.293) (-9.9323, -11.2923) (-9.9317, -11.2916) (-9.9312, -11.291) (-9.9308, -11.2906) (-9.9306, -11.2904) (-9.9304, -11.2902) (-9.9304, -11.2902) knots -1 -1 -1 -1 -1 -1 -0.99583333 -0.99166667 -0.9875 -0.98333333 -0.97916667 -0.975 -0.97083333 -0.96666667 -0.9625 -0.95833333 -0.95416667 -0.95 -0.94583333 -0.94166667 -0.9375 -0.93333333 -0.92916667 -0.925 -0.92083333 -0.91666667 -0.9125 -0.90833333 -0.90416667 -0.9 -0.89583333 -0.89166667 -0.8875 -0.88333333 -0.87916667 -0.875 -0.87083333 -0.86666667 -0.8625 -0.85833333 -0.85416667 -0.85 -0.84583333 -0.84166667 -0.8375 -0.83333333 -0.82916667 -0.825 -0.82083333 -0.81666667 -0.8125 -0.80833333 -0.80416667 -0.8 -0.79583333 -0.79166667 -0.7875 -0.78333333 -0.77916667 -0.775 -0.77083333 -0.76666667 -0.7625 -0.75833333 -0.75416667 -0.75 -0.74583333 -0.74166667 -0.7375 -0.73333333 -0.72916667 -0.725 -0.72083333 -0.71666667 -0.7125 -0.70833333 -0.70416667 -0.7 -0.69583333 -0.69166667 -0.6875 -0.68333333 -0.67916667 -0.675 -0.67083333 -0.66666667 -0.6625 -0.65833333 -0.65416667 -0.65 -0.64583333 -0.64166667 -0.6375 -0.63333333 -0.62916667 -0.625 -0.62083333 -0.61666667 -0.6125 -0.60833333 -0.60416667 -0.6 -0.59583333 -0.59166667 -0.5875 -0.58333333 -0.57916667 -0.575 -0.57083333 -0.56666667 -0.5625 -0.55833333 -0.55416667 -0.55 -0.54583333 -0.54166667 -0.5375 -0.53333333 -0.52916667 -0.525 -0.52083333 -0.51666667 -0.5125 -0.50833333 -0.50416667 -0.5 -0.49583333 -0.49166667 -0.4875 -0.48333333 -0.47916667 -0.475 -0.47083333 -0.46666667 -0.4625 -0.45833333 -0.45416667 -0.45 -0.44583333 -0.44166667 -0.4375 -0.43333333 -0.42916667 -0.425 -0.42083333 -0.41666667 -0.4125 -0.40833333 -0.40416667 -0.4 -0.39583333 -0.39166667 -0.3875 -0.38333333 -0.37916667 -0.375 -0.37083333 -0.36666667 -0.3625 -0.35833333 -0.35416667 -0.35 -0.34583333 -0.34166667 -0.3375 -0.33333333 -0.32916667 -0.325 -0.32083333 -0.31666667 -0.3125 -0.30833333 -0.30416667 -0.3 -0.29583333 -0.29166667 -0.2875 -0.28333333 -0.27916667 -0.275 -0.27083333 -0.26666667 -0.2625 -0.25833333 -0.25416667 -0.25 -0.24583333 -0.24166667 -0.2375 -0.23333333 -0.22916667 -0.225 -0.22083333 -0.21666667 -0.2125 -0.20833333 -0.20416667 -0.2 -0.19583333 -0.19166667 -0.1875 -0.18333333 -0.17916667 -0.175 -0.17083333 -0.16666667 -0.1625 -0.15833333 -0.15416667 -0.15 -0.14583333 -0.14166667 -0.1375 -0.13333333 -0.12916667 -0.125 -0.12083333 -0.11666667 -0.1125 -0.10833333 -0.10416667 -0.1 -0.09583333 -0.09166667 -0.0875 -0.08333333 -0.07916667 -0.075 -0.07083333 -0.06666667 -0.0625 -0.05833333 -0.05416667 -0.05 -0.04583333 -0.04166667 -0.0375 -0.03333333 -0.02916667 -0.025 -0.02083333 -0.01666667 -0.0125 -0.00833333 -0.00416667 0 0 0 0 0 0
  line L18 (-9.9304, -11.2902) -> (-9.9298, -11.2895)
  line L19 (-9.9298, -11.2895) -> (-9.7415, -11.0754)
  arc A10 (-9.7415, -11.0754) -> (-8.9622, -11.715) centre (0, 0) ccw
  line L20 (-8.9622, -11.715) -> (-9.1354, -11.9415)
  line L21 (-9.1354, -11.9415) -> (-9.1359, -11.9422)